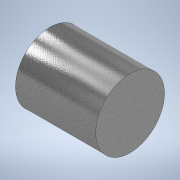
# Autodesk Inventor part: McCrea_dolny_kos_walle_MIR2
Saved by Autodesk Inventor 2022 (Build 260153000, 153)
## iProperties
Created: 2022-02-07
Part Number: McCrea_dolny_kos_walle_MIR2
Material: ABS Plastic
Document SubType Name: Modeling
Designer: student
Density: 1.06 g/cm^3
Appearance: Honed - Dark Gray
Author: student
Autodesk Inventor part; units mm, degrees
ref_plane "YZ Plane" through (0, 0, 0) normal (1, 0, 0) x (0, 1, 0)
ref_plane "XZ Plane" through (0, 0, 0) normal (0, 1, 0) x (-1, 0, 0)
ref_plane "XY Plane" through (0, 0, 0) normal (0, 0, 1) x (1, 0, 0)
sketch "Sketch1" plane through (0, 0, 0) normal (0, 0, 1) x (1, 0, 0)
  line L0 (0, 0) -> (18, 0)
  line L1 (0, 0) -> (0, 9)
  line L2 (0, 9) -> (18, 9)
  line L3 (18, 9) -> (18, 0)
  dimension "d2" = 18
  constraints: 8 end point, 1 perpendicular, 1 vertical
  measures "d2" diameter of L2 L0
revolve "Revolution1" add sketch "Sketch1" angle 360 about axis through (0, 0, 0) along (1, 0, 0)
sketch "Sketch2" plane through (0, 0, 0) normal (-1, 0, 0) x (0, 0, 1)
  circle A0 centre (0, 0) radius 8
  circle A1 centre (0, 0) radius 9 projected
  dimension "d4" = 18
  dimension "d5" = 16
  constraints: 1 centre point, 1 coincident
  measures "d4" diameter of A1
  measures "d5" diameter of A0
hole "Hole1" at (0, 0, 0) direction (1, 0, 0) diameter 16 end through all
sketch "Sketch3" plane through (18, 0, 0) normal (1, 0, 0) x (0, 0, -1)
  circle A0 centre (0, 0) radius 9
  circle A1 centre (0, 0) radius 9 projected
  dimension "d13" = 18
  dimension "d14" = 18
  constraints: 1 centre point, 1 coincident
  measures "d13" diameter of A0
  measures "d14" diameter of A1
extrude "Extrusion1" add sketch "Sketch3" along normal blind 3
sketch "Sketch4" plane through (0, 0, 0) normal (-1, 0, 0) x (0, 0, 1)
  circle A0 centre (0, 0) radius 9 projected
  circle A1 centre (0, 0) radius 8 projected
  circle A2 centre (0, 0) radius 8.5
  line L0 (0.75, -8.75) -> (-0.75, -8.75)
  line L1 (-0.75, -8.75) -> (-0.75, -8.25)
  line L2 (-0.75, -8.25) -> (0.75, -8.25)
  line L3 (0.75, -8.25) -> (0.75, -8.75)
  line L4 (8.25, -0.75) -> (8.25, 0.75)
  line L5 (8.75, -0.75) -> (8.25, -0.75)
  line L6 (8.75, 0.75) -> (8.75, -0.75)
  line L7 (8.25, 0.75) -> (8.75, 0.75)
  line L8 (0.75, 8.25) -> (-0.75, 8.25)
  line L9 (0.75, 8.75) -> (0.75, 8.25)
  line L10 (-0.75, 8.75) -> (0.75, 8.75)
  line L11 (-0.75, 8.25) -> (-0.75, 8.75)
  line L12 (-8.25, 0.75) -> (-8.25, -0.75)
  line L13 (-8.75, 0.75) -> (-8.25, 0.75)
  line L14 (-8.75, -0.75) -> (-8.75, 0.75)
  line L15 (-8.25, -0.75) -> (-8.75, -0.75)
  dimension "d17" = 18
  dimension "d18" = 17
  dimension "d19" = 0.5
  dimension "d20" = 1.5
  dimension "d21" = 0.25
  dimension "d22" = 0.75
  dimension "d26" = 360
  constraints: 32 end point, 2 parallel, 1 centre point, 1 coincident, 1 horizontal, 1 perpendicular, 33 other
  measures "d17" diameter of A0
  measures "d18" diameter of A2
  measures "d19" distance of L2.end L0.start
  measures "d20" distance of L1.end L2.end
  measures "d21" distance edge to line of A0 L0
  measures "d22" distance from line of A0.centre L3
extrude "Extrusion2" cut sketch "Sketch4" against normal blind 2 contours A2 L5 L4 L7 | A2 L7 L6 L5 | L9 L8 L11 A2 | A2 L11 L10 L9 | L3 L0 L1 A2 | A2 L1 L2 L3 | L13 L12 L15 A2 | A2 L15 L14 L13
equation "\"d6\" = d5"
equation "\"d13\" = d14"
body "Solid1"
